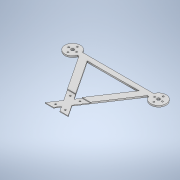
# Autodesk Inventor part: crossBraces
Saved by Autodesk Inventor 2020 (Build 240168000, 168)
## iProperties
Created: 2019-07-15
Part Number: crossBraces
Material: Generic
Document SubType Name: Modeling
Designer: Sean
Density: 1 g/cm^3
Appearance: Default
Author: Sean
Autodesk Inventor part; units mm, degrees
ref_plane "YZ Plane" through (0, 0, 0) normal (1, 0, 0) x (0, 1, 0)
ref_plane "XZ Plane" through (0, 0, 0) normal (0, 1, 0) x (-1, 0, 0)
sketch "Sketch1" plane through (0, 0, 0) normal (0, 1, 0) x (-1, 0, 0)
  circle A0 centre (0, 0) radius 3.175
  circle A1 centre (0, -9.6012) radius 1.5875
  circle A2 centre (8.1026, 0) radius 1.5875
  circle A3 centre (0, 9.6012) radius 1.5875
  circle A4 centre (-8.1026, 0) radius 1.5875
  circle A5 centre (0, 0) radius 15.875
  circle A6 centre (-176.7205, 0) radius 3.175
  circle A7 centre (-176.7332, -9.6012) radius 1.5875
  circle A8 centre (-184.8358, 0) radius 1.5875
  circle A9 centre (-176.7332, 9.6012) radius 1.5875
  circle A10 centre (-168.6306, 0) radius 1.5875
  circle A11 centre (-176.7205, 0) radius 15.875
  line L0 (-163.5506, 5.08) -> (-13.1826, 5.08)
  line L1 (-13.1826, 5.08) -> (-13.1826, -5.08)
  line L2 (-13.1826, -5.08) -> (-163.5506, -5.08)
  line L3 (-163.5506, -5.08) -> (-163.5506, 5.08)
  line L4 (0, 0) -> (-163.5506, 0)
  line L5 (-170.2181, 0) -> (-176.7078, 0)
  line L6 (-176.7205, 0) -> (-170.2181, 0)
  line L7 (-167.0431, 0) -> (-0.0127, 0)
  line L8 (-176.7078, 0) -> (-170.2181, 0)
  line L9 (-167.0431, 0) -> (-88.3666, 0)
  point P0 (-161.6802, -5.08)
  point P1 (-15.0403, -5.08)
  point P2 (-15.0403, 5.08)
  point P3 (-161.6802, 5.08)
  dimension "d0" = 6.35
  dimension "d1" = 3.175
  dimension "d2" = 3.175
  dimension "d3" = 3.175
  dimension "d4" = 3.175
  dimension "d5" = 9.6012
  dimension "d6" = 8.1026
  dimension "d7" = 8.1026
  dimension "d8" = 9.6012
  dimension "d9" = 31.75
  dimension "d14" = 5.08
  dimension "d15" = 5.08
  dimension "d16" = 5.08
  dimension "d17" = 5.08
  dimension "d50" = 176.7078
  constraints: 20 end point, 12 centre point, 4 coincident, 3 horizontal, 2 parallel, 2 point on circle, 1 midpoint, 1 perpendicular, 1 point on line
  measures "d0" diameter of A0
  measures "d1" diameter of A1
  measures "d2" diameter of A2
  measures "d3" diameter of A3
  measures "d4" diameter of A4
  measures "d5" distance of A1.centre point (0, 0)
  measures "d6" distance of point (0, 0) A2.centre
  measures "d7" distance of A4.centre point (0, 0)
  measures "d8" distance of A3.centre point (0, 0)
  measures "d9" diameter of A5
  measures "d14" distance from line of A10.centre L3
  measures "d15" distance from line of A4.centre L1
  measures "d16" distance between parallel lines of L0 L4
  measures "d17" distance between parallel lines of L2 L4
  measures "d50" distance of point (-176.72, 0) L7.end
extrude "Extrusion1" add sketch "Sketch1" along normal blind 3.048
ref_plane "Work Plane1" through (15.0403, 0, 98.425) normal (0, 0, 1) x (1, 0, 0)
mirror "Mirror1" [suppressed]
sketch "Sketch2" plane through (0, 3.048, 0) normal (0, 1, 0) x (1, 0, 0)
  arc A0 (15.0403, 5.08) -> (15.0403, -5.08) centre (0, 0) ccw projected
  line L0 (158.3147, -191.0461) -> (27.7403, 5.8039)
  arc A1 (161.6802, -5.08) -> (161.6802, 5.08) centre (176.7205, 0) ccw projected
  line L1 (18.143, -191.4206) -> (148.9802, 5.8039)
  line L2 (17.5803, -4.3561) -> (147.9282, -200.8645)
  line L3 (161.6802, -5.08) -> (159.1402, -5.08)
  line L4 (159.1402, -4.3561) -> (28.303, -201.5806)
  line L5 (95.3776, -74.9969) -> (112.2777, -74.9969)
  line L6 (81.337, -74.9969) -> (64.4377, -74.9969)
  line L7 (95.0379, -75.509) -> (111.9379, -75.509)
  line L8 (81.6767, -75.509) -> (64.7774, -75.509)
  line L9 (96.8065, -99.0548) -> (79.9064, -99.0548)
  line L10 (88.3569, -86.3038) -> (88.3569, -85.5799)
  line L11 (161.6802, 5.08) -> (15.0403, 5.08) projected
  line L12 (88.3569, -86.3038) -> (89.0808, -86.3038) construction
  line L13 (81.1864, -121.864) -> (64.2863, -121.864)
  line L14 (95.5256, -121.864) -> (112.4249, -121.864)
  line L15 (15.0403, -5.08) -> (161.6802, -5.08) projected
  line L16 (34.9598, -5.08) -> (18.0604, -5.08)
  line L17 (141.7599, -5.08) -> (159.1402, -5.08)
  point P0 (79.9068, -98.3176)
  point P1 (88.3564, -111.0559)
  point P2 (96.8065, -98.3182)
  point P3 (88.3569, -85.5799)
  point P4 (64.5631, -75.9099)
  point P5 (81.4625, -75.9099)
  point P6 (95.0379, -75.509)
  point P7 (158.66, -5.08)
  point P8 (141.7599, -5.08)
  dimension "d69" = 23.5458
  dimension "d70" = 23.5458
  dimension "d81" = 90
  dimension "d82" = 22.8092
  dimension "d83" = 22.8092
  constraints: 32 end point, 19 point on line, 5 horizontal, 3 parallel, 1 collinear, 1 perpendicular, 1 vertical, 1 other
  measures "d69" distance between parallel lines of L9 L8
  measures "d70" distance between parallel lines of L7 L9
  measures "d81" angle of L12 L10
  measures "d82" distance between parallel lines of L13 L9
  measures "d83" distance between parallel lines of L14 L9
extrude "Extrusion2" add sketch "Sketch2" against normal blind 3.048 contours L15 L0 L6 L2 | L6 L0 L8 L2 | L15 L4 L5 L1 | L5 L4 L7 L1
sketch "Sketch3" plane through (0, 0, 0) normal (0, -1, 0) x (1, 0, 0)
  line L0 (34.9598, 5.08) -> (81.6767, 75.509) projected
  line L1 (64.7774, 75.509) -> (18.0604, 5.08) projected
  line L2 (18.0604, 5.08) -> (159.8416, 218.8249)
  line L3 (15.0403, 5.08) -> (161.6802, 5.08) projected
  line L4 (34.9598, 5.08) -> (173.1628, 213.4305)
  line L5 (15.0403, 5.08) -> (161.6802, 5.08) projected
  line L6 (158.66, 5.08) -> (122.9182, 58.9573)
  line L7 (158.66, 5.08) -> (111.9379, 75.509) projected
  line L8 (158.66, 5.08) -> (25.1448, 206.3412)
  line L9 (141.7599, 5.08) -> (8.7682, 205.5521)
  line L10 (95.3776, 74.9969) -> (112.2777, 74.9969) projected
  line L11 (112.162, 75.4579) -> (95.2201, 75.4579)
  line L12 (64.4377, 74.9969) -> (81.337, 74.9969) projected
  line L13 (81.337, 75.7208) -> (64.4377, 75.7208)
  line L14 (81.675, 121.1274) -> (64.775, 121.1274)
  line L15 (111.9363, 121.1274) -> (95.037, 121.1274)
  line L16 (64.7774, 75.509) -> (81.6767, 75.509)
  line L17 (95.1415, 75.3529) -> (112.0415, 75.3529)
  line L18 (79.9064, 98.3182) -> (96.8065, 98.3182)
  point P0 (0, 0)
  point P1 (18.0604, 5.08)
  point P2 (141.7599, 5.08)
  point P3 (173.1628, 213.4305)
  point P4 (8.7682, 205.5521)
  point P5 (81.337, 74.9969)
  point P6 (88.3569, 85.5799)
  point P7 (112.2777, 74.9969)
  point P8 (96.6135, 98.7512)
  point P9 (88.3564, 111.0559)
  point P10 (79.9068, 98.3176)
  point P11 (95.3776, 74.9969)
  point P12 (81.4625, 75.9099)
  point P13 (64.5631, 75.9099)
  point P14 (111.9379, 75.509)
  dimension "d58" = 22.8092
  dimension "d64" = 22.8092
  dimension "d65" = 22.8092
  dimension "d67" = 22.9653
  constraints: 18 end point, 6 horizontal, 6 point on line, 25 other
  measures "d58" distance between parallel lines of L16 L18
  measures "d64" distance between parallel lines of L14 L18
  measures "d65" distance between parallel lines of L15 L18
  measures "d67" distance between parallel lines of L17 L18
extrude "Extrusion3" add sketch "Sketch3" against normal blind 1.524 contours L16 L2 L9 L4 | L9 L18 L4 | L4 L8 L7 L17 L9 | L8 L2 L15 L4 | L18 L2 L8 | L9 L14 L8 L2
sketch "Sketch4" plane through (0, 1.524, 0) normal (0, 1, 0) x (1, 0, 0)
  line L0 (111.9363, -121.1274) -> (96.8065, -98.3182) projected
  line L1 (79.9068, -98.3176) -> (64.775, -121.1274) projected
  line L2 (158.66, -5.08) -> (96.8065, -98.3182) projected
  line L3 (88.3564, -111.0559) -> (95.037, -121.1274) projected
  line L4 (96.8065, -98.3182) -> (88.3564, -111.0559) projected
  line L5 (96.8065, -98.3182) -> (88.3569, -85.5799) projected
  line L6 (88.3569, -85.5799) -> (88.3564, -111.0559)
  line L7 (79.9068, -98.3176) -> (88.3564, -111.0559) projected
  line L8 (96.8065, -98.3182) -> (79.9068, -98.3176)
  line L9 (88.3566, -98.3179) -> (78.3429, -83.2215)
  line L10 (88.3569, -85.5799) -> (96.8065, -98.3182) projected
  line L11 (88.3566, -98.3179) -> (98.3715, -83.2215)
  line L12 (95.0379, -75.509) -> (88.3569, -85.5799) projected
  line L13 (78.3429, -83.2215) -> (98.3715, -83.2215)
  line L14 (78.3429, -83.2215) -> (96.1304, -110.0373)
  line L15 (98.3715, -83.2215) -> (80.5501, -110.0856)
  circle A0 centre (88.3566, -98.3179) radius 18.1163
  line L16 (88.3566, -98.3179) -> (98.3708, -113.4149)
  line L17 (88.3566, -98.3179) -> (78.3425, -113.4149)
  circle A1 centre (78.3429, -83.2215) radius 1.5875
  circle A2 centre (98.3715, -83.2215) radius 1.5875
  circle A3 centre (98.3708, -113.4149) radius 1.5875
  circle A4 centre (78.3425, -113.4149) radius 1.5875
  point P0 (0, 0)
  point P1 (87.8755, -85.578)
  point P2 (87.8599, -111.6467)
  point P3 (111.9412, -75.1032)
  point P4 (64.2633, -75.4579)
  point P5 (112.162, -75.4579)
  point P6 (34.9598, -5.08)
  point P7 (18.0604, -5.08)
  point P8 (81.1626, -75.4579)
  point P9 (95.2356, -75.4579)
  point P10 (95.1415, -76.0768)
  point P11 (81.6767, -76.2329)
  point P12 (64.5631, -75.9099)
  point P13 (64.7549, -76.199)
  point P14 (112.2777, -74.9969)
  dimension "d74" = 3.175
  dimension "d75" = 3.175
  dimension "d76" = 3.175
  dimension "d77" = 3.175
  dimension "d78" = 33.559
  dimension "d79" = 33.558
  constraints: 18 end point, 5 centre point, 5 coincident, 3 point on circle, 1 horizontal, 1 midpoint, 1 point on line, 10 other
  measures "d74" diameter of A1
  measures "d75" diameter of A2
  measures "d76" diameter of A3
  measures "d77" diameter of A4
  measures "d78" angle of L6 L15
  measures "d79" angle of L6 L9
extrude "Extrusion4" cut sketch "Sketch4" against normal blind 3.81 contours A3 A0 | A0 L16 A3 | A0 A3 L16 | A2 L11 A0 | A0 A2 | A2 L13 L11 | A1 A0 L9 | L9 L13 A1 | L13 A2 A0 | A0 A1 L13 | A0 A1 | A4 A0 | A0 L17 A4 | A4 L17 A0
body "Solid1"
